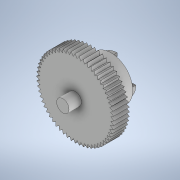
# Autodesk Inventor part: PotAttachmentB10L
Saved by Autodesk Inventor 2022 (Build 260153000, 153)
## iProperties
Created: 2021-10-23
Part Number: PotAttachmentB10L
Material: Generic
Document SubType Name: Modeling
Designer: teh18
Density: 1 g/cm^3
Appearance: Default
Author: teh18
Autodesk Inventor part; units mm, degrees
ref_plane "YZ Plane" through (0, 0, 0) normal (1, 0, 0) x (0, 1, 0)
ref_plane "XZ Plane" through (0, 0, 0) normal (0, 1, 0) x (-1, 0, 0)
ref_plane "XY Plane" through (0, 0, 0) normal (0, 0, 1) x (1, 0, 0)
sketch "Sketch1" plane through (0, 0, 0) normal (0, 0, 1) x (1, 0, 0)
  arc A0 (-0.1225, 6.9989) -> (-6, 3.6056) centre (0, 0) ccw projected
  circle A1 centre (0, 0) radius 7
  line L0 (0, -12) -> (0, -10) projected
  arc A2 (0, -10) -> (10, 0) centre (0, 0) ccw projected
  line L1 (10, 0) -> (12, 0) projected
  arc A3 (0, -12) -> (12, 0) centre (0, 0) ccw projected
  line L2 (0, 12) -> (0, 10) projected
  arc A4 (0, 10) -> (-10, 0) centre (0, 0) ccw projected
  line L3 (-10, 0) -> (-12, 0) projected
  arc A5 (0, 12) -> (-12, 0) centre (0, 0) ccw projected
  arc A6 (4.4269, -19.95) -> (6.1412, -19.4907) centre (5.1647, -19.275) ccw projected
  arc A7 (13.8088, -15.0638) -> (6.1412, -19.4907) centre (12, -20.7846) ccw projected
  arc A8 (13.8088, -15.0638) -> (15.0638, -13.8088) centre (14.1103, -14.1103) ccw projected
  arc A9 (19.4907, -6.1412) -> (15.0638, -13.8088) centre (20.7846, -12) ccw projected
  arc A10 (19.4907, -6.1412) -> (19.95, -4.4269) centre (19.275, -5.1647) ccw projected
  arc A11 (27.8571, 4.5959) -> (19.95, -4.4269) centre (24, 0) ccw projected
  arc A12 (27.8571, 4.5959) -> (29.4828, 5.5468) centre (28.5, 5.3619) ccw projected
  arc A13 (29.4828, 5.5468) -> (27.5804, 11.8035) centre (0, 0) ccw projected
  line L4 (27.5804, 11.8035) -> (33.0964, 14.1643) projected
  arc A14 (33.0964, 14.1643) -> (26.445, 24.4267) centre (0, 0) ccw projected
  line L5 (26.445, 24.4267) -> (22.0375, 20.3556) projected
  arc A15 (22.0375, 20.3556) -> (-20.3556, 22.0375) centre (0, 0) ccw projected
  line L6 (-20.3556, 22.0375) -> (-16.2845, 17.63) projected
  arc A16 (-16.2845, 17.63) -> (-5.9529, -23.25) centre (0, 0) ccw projected
  arc A17 (4.4269, -19.95) -> (-5.9529, -23.25) centre (0, -24) ccw projected
  arc A18 (-1, 6.9282) -> (-6.9282, 1) centre (0, 0) ccw projected
  line L7 (-1, 6.9282) -> (-1, 1) projected
  line L8 (-1, 1) -> (-6.9282, 1) projected
  line L9 (-6.9282, -1) -> (-1, -1) projected
  line L10 (-1, -1) -> (-1, -6.9282) projected
  arc A19 (-6.9282, -1) -> (-1, -6.9282) centre (0, 0) ccw projected
  line L11 (1, -6.9282) -> (1, -1) projected
  line L12 (1, -1) -> (6.9282, -1) projected
  arc A20 (1, -6.9282) -> (6.9282, -1) centre (0, 0) ccw projected
  line L13 (6.9282, 1) -> (1, 1) projected
  line L14 (1, 1) -> (1, 6.9282) projected
  arc A21 (6.9282, 1) -> (1, 6.9282) centre (0, 0) ccw projected
  circle A22 centre (0, 0) radius 14
  point P0 (0, 0)
  point P1 (-6, 3.6056)
  point P2 (-0.1225, 6.9989)
  dimension "d2" = 28
  constraints: 1 centre point, 1 coincident, 2 other
  measures "d2" diameter of A22
extrude "Extrusion1" add sketch "Sketch1" along normal blind 23 contours L0 A2 L1 A3 | L2 A4 L3 A5 | A22
sketch "Sketch2" plane through (0, 0, 0) normal (0, 0, -1) x (-1, 0, 0)
  line L0 (0, -12) -> (0, -10) projected
  arc A0 (-10, 0) -> (0, -10) centre (0, 0) ccw projected
  line L1 (-10, 0) -> (-12, 0) projected
  arc A1 (-12, 0) -> (0, -12) centre (0, 0) ccw projected
  line L2 (0, 12) -> (0, 10) projected
  arc A2 (10, 0) -> (0, 10) centre (0, 0) ccw projected
  line L3 (10, 0) -> (12, 0) projected
  arc A3 (12, 0) -> (0, 12) centre (0, 0) ccw projected
  arc A4 (-6.1412, -19.4907) -> (-4.4269, -19.95) centre (-5.1647, -19.275) ccw projected
  arc A5 (-6.1412, -19.4907) -> (-13.8088, -15.0638) centre (-12, -20.7846) ccw projected
  arc A6 (-15.0638, -13.8088) -> (-13.8088, -15.0638) centre (-14.1103, -14.1103) ccw projected
  arc A7 (-15.0638, -13.8088) -> (-19.4907, -6.1412) centre (-20.7846, -12) ccw projected
  arc A8 (-19.95, -4.4269) -> (-19.4907, -6.1412) centre (-19.275, -5.1647) ccw projected
  arc A9 (-19.95, -4.4269) -> (-27.8571, 4.5959) centre (-24, 0) ccw projected
  arc A10 (-29.4828, 5.5468) -> (-27.8571, 4.5959) centre (-28.5, 5.3619) ccw projected
  arc A11 (-27.5804, 11.8035) -> (-29.4828, 5.5468) centre (0, 0) ccw projected
  line L4 (-27.5804, 11.8035) -> (-33.0964, 14.1643) projected
  arc A12 (-26.445, 24.4267) -> (-33.0964, 14.1643) centre (0, 0) ccw projected
  line L5 (-26.445, 24.4267) -> (-22.0375, 20.3556) projected
  arc A13 (20.3556, 22.0375) -> (-22.0375, 20.3556) centre (0, 0) ccw projected
  line L6 (20.3556, 22.0375) -> (16.2845, 17.63) projected
  arc A14 (5.9529, -23.25) -> (16.2845, 17.63) centre (0, 0) ccw projected
  arc A15 (5.9529, -23.25) -> (-4.4269, -19.95) centre (0, -24) ccw projected
  arc A16 (6.9282, 1) -> (1, 6.9282) centre (0, 0) ccw projected
  line L7 (1, 6.9282) -> (1, 1) projected
  line L8 (1, 1) -> (6.9282, 1) projected
  line L9 (6.9282, -1) -> (1, -1) projected
  line L10 (1, -1) -> (1, -6.9282) projected
  arc A17 (1, -6.9282) -> (6.9282, -1) centre (0, 0) ccw projected
  line L11 (-1, -6.9282) -> (-1, -1) projected
  line L12 (-1, -1) -> (-6.9282, -1) projected
  arc A18 (-6.9282, -1) -> (-1, -6.9282) centre (0, 0) ccw projected
  line L13 (-6.9282, 1) -> (-1, 1) projected
  line L14 (-1, 1) -> (-1, 6.9282) projected
  arc A19 (-1, 6.9282) -> (-6.9282, 1) centre (0, 0) ccw projected
  point P0 (0, 0)
extrude "Extrusion2" add sketch "Sketch2" along normal blind 4 contours A1 L1 A0 L0 | A3 L3 A2 L2
ref_plane "Work Plane1" through (0, 0, 13) normal (0, 0, 1) x (1, 0, 0)
sketch "Sketch4" plane through (0, 0, 13) normal (0, 0, 1) x (1, 0, 0)
  circle A0 centre (0, 0) radius 3
  circle A1 centre (0, 0) radius 7 projected
  dimension "d10" = 6
  constraints: 1 centre point, 1 coincident
  measures "d10" diameter of A0
extrude "Extrusion4" add sketch "Sketch4" along normal up to surface (10 mm away) contours A0 | A1
sketch "Sketch6" plane through (0, 0, 23) normal (0, 0, 1) x (1, 0, 0)
  circle A0 centre (0, 0) radius 4
  dimension "d25" = 8
  constraints: 1 centre point, 1 coincident
  measures "d25" diameter of A0
extrude "Extrusion6" add sketch "Sketch6" along normal blind 8
sketch "Sketch7" plane through (0, 0, 13) normal (0, 0, 1) x (1, 0, 0)
  circle A0 centre (0, 0) radius 14 projected
  line L0 (0, 24.9703) -> (3, 19.7741)
  line L1 (3, 19.7741) -> (-3, 19.7741)
  line L2 (-3, 19.7741) -> (0, 24.9703)
  line L3 (-2.6101, 24.8335) -> (0.9166, 19.9794)
  line L4 (-5.0505, 19.3522) -> (-2.6101, 24.8335)
  line L5 (0.9166, 19.9794) -> (-5.0505, 19.3522)
  line L6 (-5.1916, 24.4246) -> (-1.1768, 19.9658)
  line L7 (-7.0457, 18.7183) -> (-5.1916, 24.4246)
  line L8 (-1.1768, 19.9658) -> (-7.0457, 18.7183)
  line L9 (-7.7162, 23.7482) -> (-3.2574, 19.7334)
  line L10 (-8.9637, 17.8793) -> (-7.7162, 23.7482)
  line L11 (-3.2574, 19.7334) -> (-8.9637, 17.8793)
  line L12 (-10.1563, 22.8115) -> (-5.3022, 19.2848)
  line L13 (-10.7835, 16.8444) -> (-10.1563, 22.8115)
  line L14 (-5.3022, 19.2848) -> (-10.7835, 16.8444)
  line L15 (-12.4851, 21.6249) -> (-7.289, 18.6249)
  line L16 (-12.4851, 15.6249) -> (-12.4851, 21.6249)
  line L17 (-7.289, 18.6249) -> (-12.4851, 15.6249)
  line L18 (-14.6772, 20.2014) -> (-9.1959, 17.761)
  line L19 (-14.05, 14.2343) -> (-14.6772, 20.2014)
  line L20 (-9.1959, 17.761) -> (-14.05, 14.2343)
  line L21 (-16.7084, 18.5565) -> (-11.002, 16.7024)
  line L22 (-15.4609, 12.6877) -> (-16.7084, 18.5565)
  line L23 (-11.002, 16.7024) -> (-15.4609, 12.6877)
  line L24 (-18.5565, 16.7084) -> (-12.6877, 15.4609)
  line L25 (-16.7024, 11.002) -> (-18.5565, 16.7084)
  line L26 (-12.6877, 15.4609) -> (-16.7024, 11.002)
  line L27 (-20.2014, 14.6772) -> (-14.2343, 14.05)
  line L28 (-17.761, 9.1959) -> (-20.2014, 14.6772)
  line L29 (-14.2343, 14.05) -> (-17.761, 9.1959)
  line L30 (-21.6249, 12.4851) -> (-15.6249, 12.4851)
  line L31 (-18.6249, 7.289) -> (-21.6249, 12.4851)
  line L32 (-15.6249, 12.4851) -> (-18.6249, 7.289)
  line L33 (-22.8115, 10.1563) -> (-16.8444, 10.7835)
  line L34 (-19.2848, 5.3022) -> (-22.8115, 10.1563)
  line L35 (-16.8444, 10.7835) -> (-19.2848, 5.3022)
  line L36 (-23.7482, 7.7162) -> (-17.8793, 8.9637)
  line L37 (-19.7334, 3.2574) -> (-23.7482, 7.7162)
  line L38 (-17.8793, 8.9637) -> (-19.7334, 3.2574)
  line L39 (-24.4246, 5.1916) -> (-18.7183, 7.0457)
  line L40 (-19.9658, 1.1768) -> (-24.4246, 5.1916)
  line L41 (-18.7183, 7.0457) -> (-19.9658, 1.1768)
  line L42 (-24.8335, 2.6101) -> (-19.3522, 5.0505)
  line L43 (-19.9794, -0.9166) -> (-24.8335, 2.6101)
  line L44 (-19.3522, 5.0505) -> (-19.9794, -0.9166)
  line L45 (-24.9703, 0) -> (-19.7741, 3)
  line L46 (-19.7741, -3) -> (-24.9703, 0)
  line L47 (-19.7741, 3) -> (-19.7741, -3)
  line L48 (-24.8335, -2.6101) -> (-19.9794, 0.9166)
  line L49 (-19.3522, -5.0505) -> (-24.8335, -2.6101)
  line L50 (-19.9794, 0.9166) -> (-19.3522, -5.0505)
  line L51 (-24.4246, -5.1916) -> (-19.9658, -1.1768)
  line L52 (-18.7183, -7.0457) -> (-24.4246, -5.1916)
  line L53 (-19.9658, -1.1768) -> (-18.7183, -7.0457)
  line L54 (-23.7482, -7.7162) -> (-19.7334, -3.2574)
  line L55 (-17.8793, -8.9637) -> (-23.7482, -7.7162)
  line L56 (-19.7334, -3.2574) -> (-17.8793, -8.9637)
  line L57 (-22.8115, -10.1563) -> (-19.2848, -5.3022)
  line L58 (-16.8444, -10.7835) -> (-22.8115, -10.1563)
  line L59 (-19.2848, -5.3022) -> (-16.8444, -10.7835)
  line L60 (-21.6249, -12.4851) -> (-18.6249, -7.289)
  line L61 (-15.6249, -12.4851) -> (-21.6249, -12.4851)
  line L62 (-18.6249, -7.289) -> (-15.6249, -12.4851)
  line L63 (-20.2014, -14.6772) -> (-17.761, -9.1959)
  line L64 (-14.2343, -14.05) -> (-20.2014, -14.6772)
  line L65 (-17.761, -9.1959) -> (-14.2343, -14.05)
  line L66 (-18.5565, -16.7084) -> (-16.7024, -11.002)
  line L67 (-12.6877, -15.4609) -> (-18.5565, -16.7084)
  line L68 (-16.7024, -11.002) -> (-12.6877, -15.4609)
  line L69 (-16.7084, -18.5565) -> (-15.4609, -12.6877)
  line L70 (-11.002, -16.7024) -> (-16.7084, -18.5565)
  line L71 (-15.4609, -12.6877) -> (-11.002, -16.7024)
  line L72 (-14.6772, -20.2014) -> (-14.05, -14.2343)
  line L73 (-9.1959, -17.761) -> (-14.6772, -20.2014)
  line L74 (-14.05, -14.2343) -> (-9.1959, -17.761)
  line L75 (-12.4851, -21.6249) -> (-12.4851, -15.6249)
  line L76 (-7.289, -18.6249) -> (-12.4851, -21.6249)
  line L77 (-12.4851, -15.6249) -> (-7.289, -18.6249)
  line L78 (-10.1563, -22.8115) -> (-10.7835, -16.8444)
  line L79 (-5.3022, -19.2848) -> (-10.1563, -22.8115)
  line L80 (-10.7835, -16.8444) -> (-5.3022, -19.2848)
  line L81 (-7.7162, -23.7482) -> (-8.9637, -17.8793)
  line L82 (-3.2574, -19.7334) -> (-7.7162, -23.7482)
  line L83 (-8.9637, -17.8793) -> (-3.2574, -19.7334)
  line L84 (-5.1916, -24.4246) -> (-7.0457, -18.7183)
  line L85 (-1.1768, -19.9658) -> (-5.1916, -24.4246)
  line L86 (-7.0457, -18.7183) -> (-1.1768, -19.9658)
  line L87 (-2.6101, -24.8335) -> (-5.0505, -19.3522)
  line L88 (0.9166, -19.9794) -> (-2.6101, -24.8335)
  line L89 (-5.0505, -19.3522) -> (0.9166, -19.9794)
  line L90 (0, -24.9703) -> (-3, -19.7741)
  line L91 (3, -19.7741) -> (0, -24.9703)
  line L92 (-3, -19.7741) -> (3, -19.7741)
  line L93 (2.6101, -24.8335) -> (-0.9166, -19.9794)
  line L94 (5.0505, -19.3522) -> (2.6101, -24.8335)
  line L95 (-0.9166, -19.9794) -> (5.0505, -19.3522)
  line L96 (5.1916, -24.4246) -> (1.1768, -19.9658)
  line L97 (7.0457, -18.7183) -> (5.1916, -24.4246)
  line L98 (1.1768, -19.9658) -> (7.0457, -18.7183)
  line L99 (7.7162, -23.7482) -> (3.2574, -19.7334)
  line L100 (8.9637, -17.8793) -> (7.7162, -23.7482)
  line L101 (3.2574, -19.7334) -> (8.9637, -17.8793)
  line L102 (10.1563, -22.8115) -> (5.3022, -19.2848)
  line L103 (10.7835, -16.8444) -> (10.1563, -22.8115)
  line L104 (5.3022, -19.2848) -> (10.7835, -16.8444)
  line L105 (12.4851, -21.6249) -> (7.289, -18.6249)
  line L106 (12.4851, -15.6249) -> (12.4851, -21.6249)
  line L107 (7.289, -18.6249) -> (12.4851, -15.6249)
  line L108 (14.6772, -20.2014) -> (9.1959, -17.761)
  line L109 (14.05, -14.2343) -> (14.6772, -20.2014)
  line L110 (9.1959, -17.761) -> (14.05, -14.2343)
  line L111 (16.7084, -18.5565) -> (11.002, -16.7024)
  line L112 (15.4609, -12.6877) -> (16.7084, -18.5565)
  line L113 (11.002, -16.7024) -> (15.4609, -12.6877)
  line L114 (18.5565, -16.7084) -> (12.6877, -15.4609)
  line L115 (16.7024, -11.002) -> (18.5565, -16.7084)
  line L116 (12.6877, -15.4609) -> (16.7024, -11.002)
  line L117 (20.2014, -14.6772) -> (14.2343, -14.05)
  line L118 (17.761, -9.1959) -> (20.2014, -14.6772)
  line L119 (14.2343, -14.05) -> (17.761, -9.1959)
  line L120 (21.6249, -12.4851) -> (15.6249, -12.4851)
  line L121 (18.6249, -7.289) -> (21.6249, -12.4851)
  line L122 (15.6249, -12.4851) -> (18.6249, -7.289)
  line L123 (22.8115, -10.1563) -> (16.8444, -10.7835)
  line L124 (19.2848, -5.3022) -> (22.8115, -10.1563)
  line L125 (16.8444, -10.7835) -> (19.2848, -5.3022)
  line L126 (23.7482, -7.7162) -> (17.8793, -8.9637)
  line L127 (19.7334, -3.2574) -> (23.7482, -7.7162)
  line L128 (17.8793, -8.9637) -> (19.7334, -3.2574)
  line L129 (24.4246, -5.1916) -> (18.7183, -7.0457)
  line L130 (19.9658, -1.1768) -> (24.4246, -5.1916)
  line L131 (18.7183, -7.0457) -> (19.9658, -1.1768)
  line L132 (24.8335, -2.6101) -> (19.3522, -5.0505)
  line L133 (19.9794, 0.9166) -> (24.8335, -2.6101)
  line L134 (19.3522, -5.0505) -> (19.9794, 0.9166)
  line L135 (24.9703, 0) -> (19.7741, -3)
  line L136 (19.7741, 3) -> (24.9703, 0)
  line L137 (19.7741, -3) -> (19.7741, 3)
  line L138 (24.8335, 2.6101) -> (19.9794, -0.9166)
  line L139 (19.3522, 5.0505) -> (24.8335, 2.6101)
  line L140 (19.9794, -0.9166) -> (19.3522, 5.0505)
  line L141 (24.4246, 5.1916) -> (19.9658, 1.1768)
  line L142 (18.7183, 7.0457) -> (24.4246, 5.1916)
  line L143 (19.9658, 1.1768) -> (18.7183, 7.0457)
  line L144 (23.7482, 7.7162) -> (19.7334, 3.2574)
  line L145 (17.8793, 8.9637) -> (23.7482, 7.7162)
  line L146 (19.7334, 3.2574) -> (17.8793, 8.9637)
  line L147 (22.8115, 10.1563) -> (19.2848, 5.3022)
  line L148 (16.8444, 10.7835) -> (22.8115, 10.1563)
  line L149 (19.2848, 5.3022) -> (16.8444, 10.7835)
  line L150 (21.6249, 12.4851) -> (18.6249, 7.289)
  line L151 (15.6249, 12.4851) -> (21.6249, 12.4851)
  line L152 (18.6249, 7.289) -> (15.6249, 12.4851)
  line L153 (20.2014, 14.6772) -> (17.761, 9.1959)
  line L154 (14.2343, 14.05) -> (20.2014, 14.6772)
  line L155 (17.761, 9.1959) -> (14.2343, 14.05)
  line L156 (18.5565, 16.7084) -> (16.7024, 11.002)
  line L157 (12.6877, 15.4609) -> (18.5565, 16.7084)
  line L158 (16.7024, 11.002) -> (12.6877, 15.4609)
  line L159 (16.7084, 18.5565) -> (15.4609, 12.6877)
  line L160 (11.002, 16.7024) -> (16.7084, 18.5565)
  line L161 (15.4609, 12.6877) -> (11.002, 16.7024)
  line L162 (14.6772, 20.2014) -> (14.05, 14.2343)
  line L163 (9.1959, 17.761) -> (14.6772, 20.2014)
  line L164 (14.05, 14.2343) -> (9.1959, 17.761)
  line L165 (12.4851, 21.6249) -> (12.4851, 15.6249)
  line L166 (7.289, 18.6249) -> (12.4851, 21.6249)
  line L167 (12.4851, 15.6249) -> (7.289, 18.6249)
  line L168 (10.1563, 22.8115) -> (10.7835, 16.8444)
  line L169 (5.3022, 19.2848) -> (10.1563, 22.8115)
  line L170 (10.7835, 16.8444) -> (5.3022, 19.2848)
  line L171 (7.7162, 23.7482) -> (8.9637, 17.8793)
  line L172 (3.2574, 19.7334) -> (7.7162, 23.7482)
  line L173 (8.9637, 17.8793) -> (3.2574, 19.7334)
  line L174 (5.1916, 24.4246) -> (7.0457, 18.7183)
  line L175 (1.1768, 19.9658) -> (5.1916, 24.4246)
  line L176 (7.0457, 18.7183) -> (1.1768, 19.9658)
  line L177 (2.6101, 24.8335) -> (5.0505, 19.3522)
  line L178 (-0.9166, 19.9794) -> (2.6101, 24.8335)
  line L179 (5.0505, 19.3522) -> (-0.9166, 19.9794)
  circle A1 centre (0, 0) radius 21.5062
  point P0 (0, 0)
  point P1 (0, 21.5062)
  point P2 (-2.248, 21.3884)
  point P3 (-4.4714, 21.0362)
  point P4 (-6.6458, 20.4536)
  point P5 (-8.7474, 19.6469)
  point P6 (-10.7531, 18.6249)
  point P7 (-12.641, 17.3989)
  point P8 (-14.3904, 15.9822)
  point P9 (-15.9822, 14.3904)
  point P10 (-17.3989, 12.641)
  point P11 (-18.6249, 10.7531)
  point P12 (-19.6469, 8.7474)
  point P13 (-20.4536, 6.6458)
  point P14 (-21.0362, 4.4714)
  point P15 (-21.3884, 2.248)
  point P16 (-21.5062, 0)
  point P17 (-21.3884, -2.248)
  point P18 (-21.0362, -4.4714)
  point P19 (-20.4536, -6.6458)
  point P20 (-19.6469, -8.7474)
  point P21 (-18.6249, -10.7531)
  point P22 (-17.3989, -12.641)
  point P23 (-15.9822, -14.3904)
  point P24 (-14.3904, -15.9822)
  point P25 (-12.641, -17.3989)
  point P26 (-10.7531, -18.6249)
  point P27 (-8.7474, -19.6469)
  point P28 (-6.6458, -20.4536)
  point P29 (-4.4714, -21.0362)
  point P30 (-2.248, -21.3884)
  point P31 (0, -21.5062)
  point P32 (2.248, -21.3884)
  point P33 (4.4714, -21.0362)
  point P34 (6.6458, -20.4536)
  point P35 (8.7474, -19.6469)
  point P36 (10.7531, -18.6249)
  point P37 (12.641, -17.3989)
  point P38 (14.3904, -15.9822)
  point P39 (15.9822, -14.3904)
  point P40 (17.3989, -12.641)
  point P41 (18.6249, -10.7531)
  point P42 (19.6469, -8.7474)
  point P43 (20.4536, -6.6458)
  point P44 (21.0362, -4.4714)
  point P45 (21.3884, -2.248)
  point P46 (21.5062, 0)
  point P47 (21.3884, 2.248)
  point P48 (21.0362, 4.4714)
  point P49 (20.4536, 6.6458)
  point P50 (19.6469, 8.7474)
  point P51 (18.6249, 10.7531)
  point P52 (17.3989, 12.641)
  point P53 (15.9822, 14.3904)
  point P54 (14.3904, 15.9822)
  point P55 (12.641, 17.3989)
  point P56 (10.7531, 18.6249)
  point P57 (8.7474, 19.6469)
  point P58 (6.6458, 20.4536)
  point P59 (4.4714, 21.0362)
  point P60 (2.248, 21.3884)
  point P61 (0.8332, 13.9752)
  point P62 (3.5262, 13.5487)
  point P63 (-0.6322, 13.9857)
  point P64 (2.0906, 13.843)
  point P65 (-2.0906, 13.843)
  point P66 (0.6322, 13.9857)
  point P67 (-3.5262, 13.5487)
  point P68 (-0.8332, 13.9752)
  point P69 (-4.9231, 13.1059)
  point P70 (-2.2894, 13.8115)
  point P71 (-6.266, 12.5195)
  point P72 (-3.7206, 13.4966)
  point P73 (-7.5404, 11.7959)
  point P74 (-5.111, 13.0337)
  point P75 (-8.7321, 10.9431)
  point P76 (-6.4454, 12.4281)
  point P77 (-9.8281, 9.9704)
  point P78 (-7.7091, 11.6863)
  point P79 (-10.8164, 8.8885)
  point P80 (-8.8885, 10.8164)
  point P81 (-11.6863, 7.7091)
  point P82 (-9.9704, 9.8281)
  point P83 (-12.4281, 6.4454)
  point P84 (-10.9431, 8.7321)
  point P85 (-13.0337, 5.111)
  point P86 (-11.7959, 7.5404)
  point P87 (-13.4966, 3.7206)
  point P88 (-12.5195, 6.266)
  point P89 (-13.8115, 2.2894)
  point P90 (-13.1059, 4.9231)
  point P91 (-13.9752, 0.8332)
  point P92 (-13.5487, 3.5262)
  point P93 (-13.9857, -0.6322)
  point P94 (-13.843, 2.0906)
  point P95 (-13.843, -2.0906)
  point P96 (-13.9857, 0.6322)
  point P97 (-13.5487, -3.5262)
  point P98 (-13.9752, -0.8332)
  point P99 (-13.1059, -4.9231)
  point P100 (-13.8115, -2.2894)
  point P101 (-12.5195, -6.266)
  point P102 (-13.4966, -3.7206)
  point P103 (-11.7959, -7.5404)
  point P104 (-13.0337, -5.111)
  point P105 (-10.9431, -8.7321)
  point P106 (-12.4281, -6.4454)
  point P107 (-9.9704, -9.8281)
  point P108 (-11.6863, -7.7091)
  point P109 (-8.8885, -10.8164)
  point P110 (-10.8164, -8.8885)
  point P111 (-7.7091, -11.6863)
  point P112 (-9.8281, -9.9704)
  point P113 (-6.4454, -12.4281)
  point P114 (-8.7321, -10.9431)
  point P115 (-5.111, -13.0337)
  point P116 (-7.5404, -11.7959)
  point P117 (-3.7206, -13.4966)
  point P118 (-6.266, -12.5195)
  point P119 (-2.2894, -13.8115)
  point P120 (-4.9231, -13.1059)
  point P121 (-0.8332, -13.9752)
  point P122 (-3.5262, -13.5487)
  point P123 (0.6322, -13.9857)
  point P124 (-2.0906, -13.843)
  point P125 (2.0906, -13.843)
  point P126 (-0.6322, -13.9857)
  point P127 (3.5262, -13.5487)
  point P128 (0.8332, -13.9752)
  point P129 (4.9231, -13.1059)
  point P130 (2.2894, -13.8115)
  point P131 (6.266, -12.5195)
  point P132 (3.7206, -13.4966)
  point P133 (7.5404, -11.7959)
  point P134 (5.111, -13.0337)
  point P135 (8.7321, -10.9431)
  point P136 (6.4454, -12.4281)
  point P137 (9.8281, -9.9704)
  point P138 (7.7091, -11.6863)
  point P139 (10.8164, -8.8885)
  point P140 (8.8885, -10.8164)
  point P141 (11.6863, -7.7091)
  point P142 (9.9704, -9.8281)
  point P143 (12.4281, -6.4454)
  point P144 (10.9431, -8.7321)
  point P145 (13.0337, -5.111)
  point P146 (11.7959, -7.5404)
  point P147 (13.4966, -3.7206)
  point P148 (12.5195, -6.266)
  point P149 (13.8115, -2.2894)
  point P150 (13.1059, -4.9231)
  point P151 (13.9752, -0.8332)
  point P152 (13.5487, -3.5262)
  point P153 (13.9857, 0.6322)
  point P154 (13.843, -2.0906)
  point P155 (13.843, 2.0906)
  point P156 (13.9857, -0.6322)
  point P157 (13.5487, 3.5262)
  point P158 (13.9752, 0.8332)
  point P159 (13.1059, 4.9231)
  point P160 (13.8115, 2.2894)
  point P161 (12.5195, 6.266)
  point P162 (13.4966, 3.7206)
  point P163 (11.7959, 7.5404)
  point P164 (13.0337, 5.111)
  point P165 (10.9431, 8.7321)
  point P166 (12.4281, 6.4454)
  point P167 (9.9704, 9.8281)
  point P168 (11.6863, 7.7091)
  point P169 (8.8885, 10.8164)
  point P170 (10.8164, 8.8885)
  point P171 (7.7091, 11.6863)
  point P172 (9.8281, 9.9704)
  point P173 (6.4454, 12.4281)
  point P174 (8.7321, 10.9431)
  point P175 (5.111, 13.0337)
  point P176 (7.5404, 11.7959)
  point P177 (3.7206, 13.4966)
  point P178 (6.266, 12.5195)
  point P179 (2.2894, 13.8115)
  point P180 (4.9231, 13.1059)
  point P181 (-1.0363, 19.7741)
  point P182 (1.0363, 19.7741)
  point P183 (3.0976, 19.5575)
  point P184 (5.1249, 19.1266)
  point P185 (7.0961, 18.4861)
  point P186 (8.9896, 17.6431)
  point P187 (10.7845, 16.6067)
  point P188 (12.4613, 15.3885)
  point P189 (14.0016, 14.0016)
  point P190 (15.3885, 12.4613)
  point P191 (16.6067, 10.7845)
  point P192 (17.6431, 8.9896)
  point P193 (18.4861, 7.0961)
  point P194 (19.1266, 5.1249)
  point P195 (19.5575, 3.0976)
  point P196 (19.7741, 1.0363)
  point P197 (19.7741, -1.0363)
  point P198 (19.5575, -3.0976)
  point P199 (19.1266, -5.1249)
  dimension "d28" = 6
  dimension "d31" = 360
  dimension "d36" = 2.078
  constraints: 360 end point, 2 point on line, 2 vertical alignment, 1 coincident, 1 horizontal alignment, 430 other
  measures "d28" distance of L0.end L1.end
  measures "d36" vertical distance of L0.start point (1.2, 22.892)
extrude "Extrusion7" add sketch "Sketch7" along normal up to surface (10 mm away)
sketch "Sketch5" plane through (0, 0, 13) normal (0, 0, 1) x (1, 0, 0)
  line L0 (-3, 24.9703) -> (3, 24.9703)
  line L1 (3, 24.9703) -> (3, 3)
  line L2 (3, 3) -> (-3, 3)
  line L3 (-3, 3) -> (-3, 24.9703)
  line L4 (-3, 24.9703) -> (3, 3) construction
  line L5 (3, 24.9703) -> (-3, 3) construction
  arc A0 (3, 0) -> (3, 0) centre (0, 0) ccw projected
  circle A1 centre (0, 0) radius 14 projected
  point P0 (0, 13.9851)
  point P1 (0, 24.9703)
  dimension "d14" = 6
  constraints: 12 end point, 3 midpoint, 2 parallel, 1 horizontal, 1 perpendicular
  measures "d14" distance of L1.end L2.end
extrude "Extrusion5" cut sketch "Sketch5" against normal blind 6 contours L0 L1 A1 L3 | A1 L1 L2 L3 picked at (2, 6.5583)
body "Solid1"
